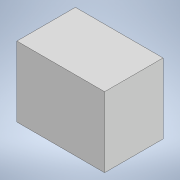
# Autodesk Inventor part: reed-switch-design-test
Saved by Autodesk Inventor 2021 (Build 250183000, 183)
## iProperties
Created: 2021-01-14
Part Number: reed-switch-design-test
Material: Generic
Document SubType Name: Modeling
Designer: Luke Kamols
Density: 1 g/cm^3
Appearance: Default
Author: Luke Kamols
Autodesk Inventor part; units mm, degrees
ref_plane "YZ Plane" through (0, 0, 0) normal (1, 0, 0) x (0, 1, 0)
ref_plane "XZ Plane" through (0, 0, 0) normal (0, 1, 0) x (-1, 0, 0)
ref_plane "XY Plane" through (0, 0, 0) normal (0, 0, 1) x (1, 0, 0)
sketch "Sketch3" plane through (0, 0, 0) normal (0, 1, 0) x (-1, 0, 0)
  line L0 (0, 0) -> (9, 0)
  line L1 (9, 0) -> (9, -3)
  line L2 (9, -3) -> (0, -3)
  line L3 (0, -3) -> (0, 0)
  line L4 (0, 1) -> (12, 1)
  line L5 (12, 1) -> (12, -9)
  line L6 (12, -9) -> (-3, -9)
  line L7 (0, 1) -> (-3, 1)
  line L8 (-3, 1) -> (-3, -9)
  dimension "d17" = 3
  dimension "d19" = 12
  dimension "d20" = 10
  constraints: 18 end point, 6 perpendicular, 2 horizontal, 1 parallel
  measures "d17" distance of L0.end L1.end
  measures "d19" distance of L4.start L4.end
  measures "d20" distance of L4.end L5.end
extrude "Extrusion3" add sketch "Sketch3" along normal blind 10
sketch "Sketch4" plane through (0, 10, 0) normal (0, 1, 0) x (1, 0, 0)
  line L0 (-12, 9) -> (-12, -1) projected
  line L1 (3, 9) -> (-12, 9) projected
  line L2 (3, -1) -> (3, 9) projected
  line L3 (-12, -1) -> (3, -1) projected
  point P0 (0, 0)
extrude "Extrusion4" add sketch "Sketch4" along normal blind 2
body "Solid2"
